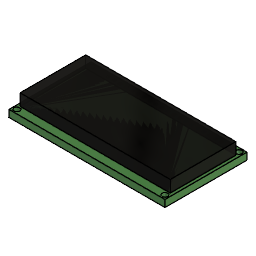
Screen for PCB footprint v2 (Autodesk Fusion 360 design; units mm, degrees)
Autodesk Fusion 360 part; units mm, degrees
sketch "Sketch4" plane through (0, 0, 0) normal (0, 0, 1) x (1, 0, 0)
  line L0 (33.25, -17.5) -> (-33.25, -17.5)
  line L1 (-33.25, -17.5) -> (-33.25, 17.5)
  line L2 (-33.25, 17.5) -> (33.25, 17.5)
  line L3 (33.25, 17.5) -> (33.25, -17.5)
  line L4 (33.25, -17.5) -> (-33.25, 17.5) construction
  line L5 (-33.25, -17.5) -> (33.25, 17.5) construction
  dimension "d17" = 66.5
  dimension "d18" = 35
  constraint horizontal L0
  constraint perpendicular L0 L1
  constraint parallel L0 L2
  constraint parallel L1 L3
  constraint coincident L4 origin
  constraint coincident L5 origin
  measures "d17" distance of L0.start L0.end
  measures "d18" distance of L0.end L1.end
extrude "Extrude3" add sketch "Sketch4" along normal blind 3 makes body 1
sketch "Sketch5" plane through (0, 0, 3) normal (0, 0, 1) x (-1, 0, 0)
  line L0 (-33.25, -17.5) -> (33.25, -17.5)
  line L1 (33.25, -17.5) -> (33.25, 17.5)
  line L2 (33.25, 17.5) -> (-33.25, 17.5)
  line L3 (-33.25, 17.5) -> (-33.25, -17.5)
  line L4 (-32, 14) -> (32, 14)
  line L5 (32, 14) -> (32, -14)
  line L6 (32, -14) -> (-32, -14)
  line L7 (-32, -14) -> (-32, 14)
  line L8 (-32, 14) -> (32, -14) construction
  line L9 (32, 14) -> (-32, -14) construction
  circle A0 centre (31.55, -15.8) radius 1.2
  line L10 (0, 17.5) -> (0, -17.5) construction
  line L11 (-33.25, 0) -> (33.25, 0) construction
  line L12 (0.92, -15.15) -> (1.62, -15.15)
  line L13 (1.77, -15.3) -> (1.77, -16.2)
  line L14 (1.62, -16.35) -> (0.92, -16.35)
  line L15 (0.77, -16.2) -> (0.77, -15.3)
  circle A1 centre (-31.55, -15.8) radius 1.2
  circle A2 centre (31.55, 15.8) radius 1.2
  circle A3 centre (-31.55, 15.8) radius 1.2
  arc A4 (1.62, -16.35) -> (1.77, -16.2) centre (1.62, -16.2) ccw
  arc A5 (0.77, -16.2) -> (0.92, -16.35) centre (0.92, -16.2) ccw
  arc A6 (0.92, -15.15) -> (0.77, -15.3) centre (0.92, -15.3) ccw
  arc A7 (1.77, -15.3) -> (1.62, -15.15) centre (1.62, -15.3) ccw
  line L16 (4.31, -15.3) -> (4.31, -16.2)
  line L17 (4.16, -16.35) -> (3.46, -16.35)
  arc A8 (3.46, -15.15) -> (3.31, -15.3) centre (3.46, -15.3) ccw
  line L18 (3.31, -16.2) -> (3.31, -15.3)
  line L19 (3.46, -15.15) -> (4.16, -15.15)
  arc A9 (4.31, -15.3) -> (4.16, -15.15) centre (4.16, -15.3) ccw
  arc A10 (4.16, -16.35) -> (4.31, -16.2) centre (4.16, -16.2) ccw
  arc A11 (3.31, -16.2) -> (3.46, -16.35) centre (3.46, -16.2) ccw
  line L20 (6.85, -15.3) -> (6.85, -16.2)
  line L21 (6.7, -16.35) -> (6, -16.35)
  arc A12 (6, -15.15) -> (5.85, -15.3) centre (6, -15.3) ccw
  line L22 (5.85, -16.2) -> (5.85, -15.3)
  line L23 (6, -15.15) -> (6.7, -15.15)
  arc A13 (6.85, -15.3) -> (6.7, -15.15) centre (6.7, -15.3) ccw
  arc A14 (6.7, -16.35) -> (6.85, -16.2) centre (6.7, -16.2) ccw
  arc A15 (5.85, -16.2) -> (6, -16.35) centre (6, -16.2) ccw
  line L24 (9.39, -15.3) -> (9.39, -16.2)
  line L25 (9.24, -16.35) -> (8.54, -16.35)
  arc A16 (8.54, -15.15) -> (8.39, -15.3) centre (8.54, -15.3) ccw
  line L26 (8.39, -16.2) -> (8.39, -15.3)
  line L27 (8.54, -15.15) -> (9.24, -15.15)
  arc A17 (9.39, -15.3) -> (9.24, -15.15) centre (9.24, -15.3) ccw
  arc A18 (9.24, -16.35) -> (9.39, -16.2) centre (9.24, -16.2) ccw
  arc A19 (8.39, -16.2) -> (8.54, -16.35) centre (8.54, -16.2) ccw
  line L28 (11.93, -15.3) -> (11.93, -16.2)
  line L29 (11.78, -16.35) -> (11.08, -16.35)
  arc A20 (11.08, -15.15) -> (10.93, -15.3) centre (11.08, -15.3) ccw
  line L30 (10.93, -16.2) -> (10.93, -15.3)
  line L31 (11.08, -15.15) -> (11.78, -15.15)
  arc A21 (11.93, -15.3) -> (11.78, -15.15) centre (11.78, -15.3) ccw
  arc A22 (11.78, -16.35) -> (11.93, -16.2) centre (11.78, -16.2) ccw
  arc A23 (10.93, -16.2) -> (11.08, -16.35) centre (11.08, -16.2) ccw
  line L32 (14.47, -15.3) -> (14.47, -16.2)
  line L33 (14.32, -16.35) -> (13.62, -16.35)
  arc A24 (13.62, -15.15) -> (13.47, -15.3) centre (13.62, -15.3) ccw
  line L34 (13.47, -16.2) -> (13.47, -15.3)
  line L35 (13.62, -15.15) -> (14.32, -15.15)
  arc A25 (14.47, -15.3) -> (14.32, -15.15) centre (14.32, -15.3) ccw
  arc A26 (14.32, -16.35) -> (14.47, -16.2) centre (14.32, -16.2) ccw
  arc A27 (13.47, -16.2) -> (13.62, -16.35) centre (13.62, -16.2) ccw
  line L36 (17.01, -15.3) -> (17.01, -16.2)
  line L37 (16.86, -16.35) -> (16.16, -16.35)
  arc A28 (16.16, -15.15) -> (16.01, -15.3) centre (16.16, -15.3) ccw
  line L38 (16.01, -16.2) -> (16.01, -15.3)
  line L39 (16.16, -15.15) -> (16.86, -15.15)
  arc A29 (17.01, -15.3) -> (16.86, -15.15) centre (16.86, -15.3) ccw
  arc A30 (16.86, -16.35) -> (17.01, -16.2) centre (16.86, -16.2) ccw
  arc A31 (16.01, -16.2) -> (16.16, -16.35) centre (16.16, -16.2) ccw
  line L40 (19.55, -15.3) -> (19.55, -16.2)
  line L41 (19.4, -16.35) -> (18.7, -16.35)
  arc A32 (18.7, -15.15) -> (18.55, -15.3) centre (18.7, -15.3) ccw
  line L42 (18.55, -16.2) -> (18.55, -15.3)
  line L43 (18.7, -15.15) -> (19.4, -15.15)
  arc A33 (19.55, -15.3) -> (19.4, -15.15) centre (19.4, -15.3) ccw
  arc A34 (19.4, -16.35) -> (19.55, -16.2) centre (19.4, -16.2) ccw
  arc A35 (18.55, -16.2) -> (18.7, -16.35) centre (18.7, -16.2) ccw
  line L44 (22.09, -15.3) -> (22.09, -16.2)
  line L45 (21.94, -16.35) -> (21.24, -16.35)
  arc A36 (21.24, -15.15) -> (21.09, -15.3) centre (21.24, -15.3) ccw
  line L46 (21.09, -16.2) -> (21.09, -15.3)
  line L47 (21.24, -15.15) -> (21.94, -15.15)
  arc A37 (22.09, -15.3) -> (21.94, -15.15) centre (21.94, -15.3) ccw
  arc A38 (21.94, -16.35) -> (22.09, -16.2) centre (21.94, -16.2) ccw
  arc A39 (21.09, -16.2) -> (21.24, -16.35) centre (21.24, -16.2) ccw
  line L48 (24.63, -15.3) -> (24.63, -16.2)
  line L49 (24.48, -16.35) -> (23.78, -16.35)
  arc A40 (23.78, -15.15) -> (23.63, -15.3) centre (23.78, -15.3) ccw
  line L50 (23.63, -16.2) -> (23.63, -15.3)
  line L51 (23.78, -15.15) -> (24.48, -15.15)
  arc A41 (24.63, -15.3) -> (24.48, -15.15) centre (24.48, -15.3) ccw
  arc A42 (24.48, -16.35) -> (24.63, -16.2) centre (24.48, -16.2) ccw
  arc A43 (23.63, -16.2) -> (23.78, -16.35) centre (23.78, -16.2) ccw
  arc A44 (-6.85, -16.2) -> (-6.7, -16.35) centre (-6.7, -16.2) ccw
  arc A45 (-1.62, -15.15) -> (-1.77, -15.3) centre (-1.62, -15.3) ccw
  line L52 (-16.86, -16.35) -> (-16.16, -16.35)
  line L53 (-19.55, -15.3) -> (-19.55, -16.2)
  line L54 (-5.85, -16.2) -> (-5.85, -15.3)
  arc A46 (-21.94, -15.15) -> (-22.09, -15.3) centre (-21.94, -15.3) ccw
  line L55 (-22.09, -15.3) -> (-22.09, -16.2)
  line L56 (-9.39, -15.3) -> (-9.39, -16.2)
  line L57 (-3.31, -16.2) -> (-3.31, -15.3)
  arc A47 (-19.4, -15.15) -> (-19.55, -15.3) centre (-19.4, -15.3) ccw
  line L58 (-8.54, -15.15) -> (-9.24, -15.15)
  line L59 (-1.62, -16.35) -> (-0.92, -16.35)
  arc A48 (-9.39, -16.2) -> (-9.24, -16.35) centre (-9.24, -16.2) ccw
  line L60 (-9.24, -16.35) -> (-8.54, -16.35)
  line L61 (-11.78, -16.35) -> (-11.08, -16.35)
  arc A49 (-6.7, -15.15) -> (-6.85, -15.3) centre (-6.7, -15.3) ccw
  arc A50 (-9.24, -15.15) -> (-9.39, -15.3) centre (-9.24, -15.3) ccw
  line L62 (-6.85, -15.3) -> (-6.85, -16.2)
  line L63 (-18.7, -15.15) -> (-19.4, -15.15)
  arc A51 (-8.39, -15.3) -> (-8.54, -15.15) centre (-8.54, -15.3) ccw
  line L64 (-10.93, -16.2) -> (-10.93, -15.3)
  arc A52 (-4.31, -16.2) -> (-4.16, -16.35) centre (-4.16, -16.2) ccw
  arc A53 (-14.47, -16.2) -> (-14.32, -16.35) centre (-14.32, -16.2) ccw
  arc A54 (-21.24, -16.35) -> (-21.09, -16.2) centre (-21.24, -16.2) ccw
  arc A55 (-17.01, -16.2) -> (-16.86, -16.35) centre (-16.86, -16.2) ccw
  line L65 (-21.94, -16.35) -> (-21.24, -16.35)
  arc A56 (-24.48, -15.15) -> (-24.63, -15.3) centre (-24.48, -15.3) ccw
  line L66 (-21.09, -16.2) -> (-21.09, -15.3)
  arc A57 (-13.62, -16.35) -> (-13.47, -16.2) centre (-13.62, -16.2) ccw
  line L67 (-0.77, -16.2) -> (-0.77, -15.3)
  line L68 (-17.01, -15.3) -> (-17.01, -16.2)
  arc A58 (-0.77, -15.3) -> (-0.92, -15.15) centre (-0.92, -15.3) ccw
  line L69 (-1.77, -15.3) -> (-1.77, -16.2)
  arc A59 (-13.47, -15.3) -> (-13.62, -15.15) centre (-13.62, -15.3) ccw
  line L70 (-21.24, -15.15) -> (-21.94, -15.15)
  line L71 (-24.63, -15.3) -> (-24.63, -16.2)
  line L72 (-19.4, -16.35) -> (-18.7, -16.35)
  arc A60 (-10.93, -15.3) -> (-11.08, -15.15) centre (-11.08, -15.3) ccw
  arc A61 (-21.09, -15.3) -> (-21.24, -15.15) centre (-21.24, -15.3) ccw
  arc A62 (-24.63, -16.2) -> (-24.48, -16.35) centre (-24.48, -16.2) ccw
  arc A63 (-18.55, -15.3) -> (-18.7, -15.15) centre (-18.7, -15.3) ccw
  arc A64 (-11.93, -16.2) -> (-11.78, -16.35) centre (-11.78, -16.2) ccw
  arc A65 (-23.78, -16.35) -> (-23.63, -16.2) centre (-23.78, -16.2) ccw
  line L73 (-16.16, -15.15) -> (-16.86, -15.15)
  arc A66 (-16.01, -15.3) -> (-16.16, -15.15) centre (-16.16, -15.3) ccw
  line L74 (-16.01, -16.2) -> (-16.01, -15.3)
  line L75 (-23.78, -15.15) -> (-24.48, -15.15)
  line L76 (-11.93, -15.3) -> (-11.93, -16.2)
  line L77 (-24.48, -16.35) -> (-23.78, -16.35)
  arc A67 (-16.16, -16.35) -> (-16.01, -16.2) centre (-16.16, -16.2) ccw
  arc A68 (-16.86, -15.15) -> (-17.01, -15.3) centre (-16.86, -15.3) ccw
  arc A69 (-19.55, -16.2) -> (-19.4, -16.35) centre (-19.4, -16.2) ccw
  arc A70 (-18.7, -16.35) -> (-18.55, -16.2) centre (-18.7, -16.2) ccw
  line L78 (-11.08, -15.15) -> (-11.78, -15.15)
  line L79 (-13.62, -15.15) -> (-14.32, -15.15)
  arc A71 (-3.31, -15.3) -> (-3.46, -15.15) centre (-3.46, -15.3) ccw
  arc A72 (-3.46, -16.35) -> (-3.31, -16.2) centre (-3.46, -16.2) ccw
  line L80 (-23.63, -16.2) -> (-23.63, -15.3)
  line L81 (-14.32, -16.35) -> (-13.62, -16.35)
  arc A73 (-6, -16.35) -> (-5.85, -16.2) centre (-6, -16.2) ccw
  arc A74 (-5.85, -15.3) -> (-6, -15.15) centre (-6, -15.3) ccw
  line L82 (-8.39, -16.2) -> (-8.39, -15.3)
  arc A75 (-1.77, -16.2) -> (-1.62, -16.35) centre (-1.62, -16.2) ccw
  arc A76 (-11.08, -16.35) -> (-10.93, -16.2) centre (-11.08, -16.2) ccw
  arc A77 (-4.16, -15.15) -> (-4.31, -15.3) centre (-4.16, -15.3) ccw
  line L83 (-4.31, -15.3) -> (-4.31, -16.2)
  arc A78 (-8.54, -16.35) -> (-8.39, -16.2) centre (-8.54, -16.2) ccw
  arc A79 (-14.32, -15.15) -> (-14.47, -15.3) centre (-14.32, -15.3) ccw
  line L84 (-0.92, -15.15) -> (-1.62, -15.15)
  line L85 (-14.47, -15.3) -> (-14.47, -16.2)
  line L86 (-6, -15.15) -> (-6.7, -15.15)
  arc A80 (-23.63, -15.3) -> (-23.78, -15.15) centre (-23.78, -15.3) ccw
  arc A81 (-22.09, -16.2) -> (-21.94, -16.35) centre (-21.94, -16.2) ccw
  line L87 (-3.46, -15.15) -> (-4.16, -15.15)
  arc A82 (-0.92, -16.35) -> (-0.77, -16.2) centre (-0.92, -16.2) ccw
  line L88 (-6.7, -16.35) -> (-6, -16.35)
  line L89 (-18.55, -16.2) -> (-18.55, -15.3)
  line L90 (-4.16, -16.35) -> (-3.46, -16.35)
  arc A83 (-11.78, -15.15) -> (-11.93, -15.3) centre (-11.78, -15.3) ccw
  line L91 (-13.47, -16.2) -> (-13.47, -15.3)
  dimension "d21" = 64
  dimension "d22" = 28
  dimension "d23" = 2.4
  dimension "d24" = 1.7
  dimension "d25" = 1.7
  dimension "d45" = 1.2
  dimension "d46" = 1
  dimension "d47" = 0.15
  dimension "d48" = 0.15
  dimension "d49" = 0.15
  dimension "d50" = 0.15
  dimension "d51" = 0.15
  dimension "d52" = 0.15
  dimension "d53" = 0.15
  dimension "d54" = 0.15
  dimension "d55" = 1.15
  dimension "d56" = 0.77
  dimension "d59" = 22.86
  dimension "d60" = 0
  constraint horizontal L4
  constraint perpendicular L4 L5
  constraint parallel L4 L6
  constraint parallel L5 L7
  constraint coincident L8 origin
  constraint coincident L9 origin
  constraint midpoint L2 L10.start
  constraint midpoint L0 L10.end
  constraint midpoint L3 L11.start
  constraint midpoint L1 L11.end
  constraint horizontal L12
  constraint perpendicular L12 L13
  constraint parallel L12 L14
  constraint parallel L13 L15
  constraint symmetric A0 L10 A1
  constraint symmetric A0 L11 A2
  constraint symmetric L11 A1 A3
  constraint tangent L13 A4
  constraint tangent L15 A5
  constraint tangent L12 A6
  constraint tangent L12 A7
  constraint symmetric L10 L13.end L69.end
  constraint symmetric L10 L14.start L59.start
  constraint symmetric L10 A4 A75
  constraint symmetric L10 L14.end L59.end
  constraint symmetric L10 L15.start L67.start
  constraint symmetric L10 A5 A82
  constraint symmetric L10 L15.end L67.end
  constraint symmetric L10 L12.start A58.end
  constraint symmetric L10 A6 A58
  constraint symmetric L10 L12.end A45.start
  constraint symmetric L10 L13.start A45.end
  constraint symmetric L10 A7 A45
  constraint symmetric L10 A8.end L57.end
  constraint symmetric L10 L16.end A52.start
  constraint symmetric L10 L16.start A77.end
  constraint symmetric L10 L17.start A52.end
  constraint symmetric L10 L17.end A72.start
  constraint symmetric L10 L19.end A77.start
  constraint symmetric L10 A8.start A71.end
  constraint symmetric L10 A8 A71
  constraint symmetric L10 L18.start L57.start
  constraint symmetric L10 A9 A77
  constraint symmetric L10 A10 A52
  constraint symmetric L10 A11 A72
  constraint symmetric L10 A12.end L54.end
  constraint symmetric L10 L20.end A44.start
  constraint symmetric L10 L20.start A49.end
  constraint symmetric L10 L21.start A44.end
  constraint symmetric L10 L21.end A73.start
  constraint symmetric L10 L23.end A49.start
  constraint symmetric L10 A12.start A74.end
  constraint symmetric L10 A12 A74
  constraint symmetric L10 L22.start L54.start
  constraint symmetric L10 A13 A49
  constraint symmetric L10 A14 A44
  constraint symmetric L10 A15 A73
  constraint symmetric L10 A16.end A51.start
  constraint symmetric L10 L24.end L56.end
  constraint symmetric L10 L24.start L56.start
  constraint symmetric L10 L25.start A48.end
  constraint symmetric L10 L25.end L60.end
  constraint symmetric L10 L27.end L58.end
  constraint symmetric L10 A16.start L58.start
  constraint symmetric L10 A16 A51
  constraint symmetric L10 L26.start L82.start
  constraint symmetric L10 A17 A50
  constraint symmetric L10 A18 A48
  constraint symmetric L10 A19 A78
  constraint symmetric L10 A20.end L64.end
  constraint symmetric L10 L28.end A64.start
  constraint symmetric L10 L28.start L76.start
  constraint symmetric L10 L29.start L61.start
  constraint symmetric L10 L29.end L61.end
  constraint symmetric L10 L31.end L78.end
  constraint symmetric L10 A20.start A60.end
  constraint symmetric L10 A20 A60
  constraint symmetric L10 L30.start L64.start
  constraint symmetric L10 A21 A83
  constraint symmetric L10 A22 A64
  constraint symmetric L10 A23 A76
  constraint symmetric L10 A24.end A59.start
  constraint symmetric L10 L32.end A53.start
  constraint symmetric L10 L32.start A79.end
  constraint symmetric L10 L33.start A53.end
  constraint symmetric L10 L33.end A57.start
  constraint symmetric L10 L35.end L79.end
  constraint symmetric L10 A24.start A59.end
  constraint symmetric L10 A24 A59
  constraint symmetric L10 L34.start A57.end
  constraint symmetric L10 A25 A79
  constraint symmetric L10 A26 A53
  constraint symmetric L10 A27 A57
  constraint symmetric L10 A28.end A66.start
  constraint symmetric L10 L36.end A55.start
  constraint symmetric L10 L36.start L68.start
  constraint symmetric L10 L37.start L52.start
  constraint symmetric L10 L37.end L52.end
  constraint symmetric L10 L39.end L73.end
  constraint symmetric L10 A28.start L73.start
  constraint symmetric L10 A28 A66
  constraint symmetric L10 L38.start L74.start
  constraint symmetric L10 A29 A68
  constraint symmetric L10 A30 A55
  constraint symmetric L10 A31 A67
  constraint symmetric L10 A32.end A63.start
  constraint symmetric L10 L40.end L53.end
  constraint symmetric L10 L40.start L53.start
  constraint symmetric L10 L41.start L72.start
  constraint symmetric L10 L41.end L72.end
  constraint symmetric L10 L43.end A47.start
  constraint symmetric L10 A32.start L63.start
  constraint symmetric L10 A32 A63
  constraint symmetric L10 L42.start A70.end
  constraint symmetric L10 A33 A47
  constraint symmetric L10 A34 A69
  constraint symmetric L10 A35 A70
  constraint symmetric L10 A36.end L66.end
  constraint symmetric L10 L44.end L55.end
  constraint symmetric L10 L44.start A46.end
  constraint symmetric L10 L45.start L65.start
  constraint symmetric L10 L45.end A54.start
  constraint symmetric L10 L47.end A46.start
  constraint symmetric L10 A36.start L70.start
  constraint symmetric L10 A36 A61
  constraint symmetric L10 L46.start A54.end
  constraint symmetric L10 A37 A46
  constraint symmetric L10 A38 A81
  constraint symmetric L10 A39 A54
  constraint symmetric L10 A40.end L80.end
  constraint symmetric L10 L48.end L71.end
  constraint symmetric L10 L48.start A56.end
  constraint symmetric L10 L49.start A62.end
  constraint symmetric L10 L49.end A65.start
  constraint symmetric L10 L51.end A56.start
  constraint symmetric L10 A40.start L75.start
  constraint symmetric L10 A40 A80
  constraint symmetric L10 L50.start A65.end
  constraint symmetric L10 A41 A56
  constraint symmetric L10 A42 A62
  constraint symmetric L10 A43 A65
  measures "d21" distance of L4.start L4.end
  measures "d22" distance of L4.start L6.end
  measures "d23" diameter of A0
  measures "d24" distance of L0 A0.centre
  measures "d25" distance of L1 A0.centre
  measures "d45" distance of L12 L14
  measures "d46" distance of L13 L15
  measures "d47" distance of L15 A5.centre
  measures "d48" distance of L14 A5.centre
  measures "d49" distance of L14 A4.centre
  measures "d50" distance of L13 A4.centre
  measures "d51" distance of L13 A7.centre
  measures "d52" distance of L12 A7.centre
  measures "d53" distance of L12 A6.centre
  measures "d54" distance of L15 A6.centre
  measures "d55" distance of L0 L14
  measures "d56" distance of L10 L15
extrude "Extrude4" cut sketch "Sketch5" against normal through all contours A0 | L12 L13 L14 L15 A4 A5 A6 A7 | A1 | A2 | A3 | L16 L17 A8 L18 L19 A9 A10 A11 | L20 L21 A12 L22 L23 A13 A14 A15 | L24 L25 A16 L26 L27 A17 A18 A19 | L28 L29 A20 L30 L31 A21 A22 A23 | L32 L33 A24 L34 L35 A25 A26 A27 | L36 L37 A28 L38 L39 A29 A30 A31 | L40 L41 A32 L42 L43 A33 A34 A35 | L44 L45 A36 L46 L47 A37 A38 A39 | L48 L49 A40 L50 L51 A41 A42 A43 | A44 L54 A49 L62 A73 A74 L86 L88 | A45 L59 L67 A58 L69 A75 L84 A82 | L52 A55 L68 L73 A66 L74 A67 A68 | L53 A47 L63 L72 A63 A69 A70 L89 | A46 L55 A54 L65 L66 L70 A61 A81 | L56 L58 A48 L60 A50 A51 L82 A78 | L57 A52 A71 A72 A77 L83 L87 L90 | L61 L64 A60 A64 L76 L78 A76 A83 | A53 A57 A59 L79 L81 A79 L85 L91 | A56 L71 A62 A65 L75 L77 L80 A80 bodies 1
extrude "Extrude5" add sketch "Sketch5" along normal blind 5 separate body contours L4 L5 L6 L7 makes body 2
